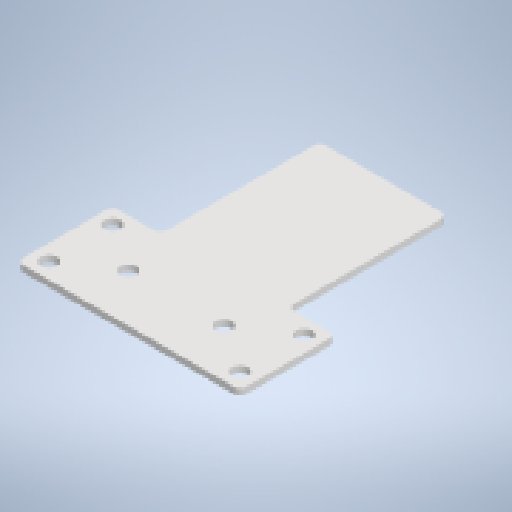
# Autodesk Inventor part: NDM 11.030 plate
Saved by Autodesk Inventor 2025 (Build 290162010, 162A)
## iProperties
Created: 2024-06-12
Part Number: NDM 11.030 plate
Material: Stainless Steel
Document SubType Name: Sheet Metal
Designer: admin
Density: 8 g/cm^3
Flat Pattern Width: 7 cm
Flat Pattern Length: 8 cm
Flat Pattern Area: 56 cm^2
Sheet Metal Rule: AISI304 2mm Die16
Sheet Metal Width: 70,000 mm
Sheet Metal Length: 80,000 mm
Sheet Metal Area: 5600,000 mm^2
Appearance: Default
Mass: 55.3167 g
Surface Area: 74.8369 cm^2
Volume: 6.91459 cm^3
Description: 2mm
Author: admin
Revision Number: 20
Autodesk Inventor part; units mm, degrees
ref_plane "YZ Plane" through (0, 0, 0) normal (1, 0, 0) x (0, 1, 0)
ref_plane "XZ Plane" through (0, 0, 0) normal (0, 1, 0) x (-1, 0, 0)
ref_plane "XY Plane" through (0, 0, 0) normal (0, 0, 1) x (1, 0, 0)
sketch "Sketch1" plane through (0, 0, 0) normal (0, 0, 1) x (1, 0, 0)
  line L0 (-20, 0) -> (20, 0)
  line L1 (20, 0) -> (20, -50)
  line L2 (20, -50) -> (-20, -50)
  line L3 (-20, -50) -> (-20, 0)
  line L4 (-35, -80) -> (35, -80)
  line L5 (35, -80) -> (35, -50)
  line L6 (35, -50) -> (-35, -50)
  line L7 (-35, -50) -> (-35, -80)
  circle A0 centre (-15, -65) radius 2.5
  circle A1 centre (15, -65) radius 2.5
  line L8 (0, -80) -> (0, -50) construction
  circle A2 centre (-30, -55) radius 2.5
  circle A3 centre (30, -55) radius 2.5
  circle A4 centre (30, -75) radius 2.5
  circle A5 centre (-30, -75) radius 2.5
  line L9 (-35, -65) -> (35, -65) construction
  point P0 (0, 0)
  point P1 (0, 0)
  dimension "d0" = 40
  dimension "d1" = 50
  dimension "d33" = 70
  dimension "d34" = 5
  dimension "d35" = 30
  dimension "d36" = 30
  dimension "d38" = 5
  dimension "d39" = 5
  measures "d0" distance of L1.end L2.end
  measures "d1" distance of L0.end L1.end
  measures "d33" distance between parallel lines of L5 L7
  measures "d34" diameter of A1
  measures "d35" distance of A0.centre A1.centre
  measures "d36" distance of L4.end L5.end
  measures "d38" distance from line of L4 A5.centre
  measures "d39" distance from line of A5.centre L7
extrude "Plate1" add sketch "Sketch1" along normal blind 2
fillet "Corner Round1" radius 2 8 edges at (-20, -50, 1) (-35, -50, 1) (20, -50, 1) (35, -50, 1) (35, -80, 1) (-35, -80, 1) (-20, 0, 1) (20, 0, 1)
equation "\"d2\" = Thickness"
equation "\"BendReliefWidth\" = Thickness"
equation "\"BendReliefDepth\" = 0.5 * Thickness"
equation "\"CornerReliefSize\" = 4 * Thickness"
equation "\"MinimumRemnant\" = 2 * Thickness"
equation "\"TransitionRadius\" = BendRadius"
equation "\"JacobiRadiusSize\" = BendRadius"
equation "\"GapSize\" = Thickness"
equation "\"Thickness\" = 2"
equation "\"BendRadius\" = 2.75"
body "Solid1"
